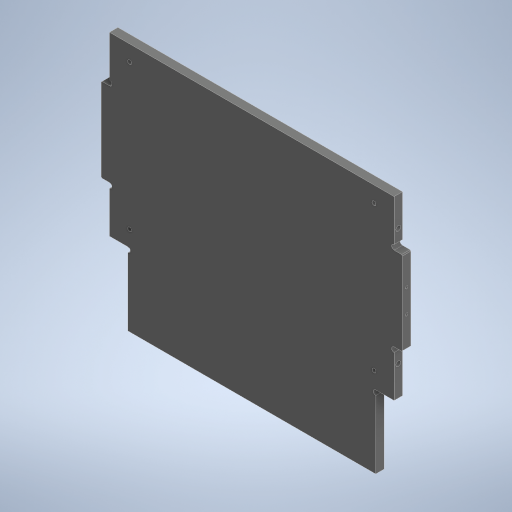
# Autodesk Inventor part: TorsoCoverFrameBasis
Saved by Autodesk Inventor 2024.2 (Build 282272000, 272)
## iProperties
Created: 2024-01-05
Part Number: TorsoCoverFrameBasis
Material: Acetal Resin, Black
Document SubType Name: Modeling
Designer: Masato Kubotera
Density: 1.425 g/cm^3
Appearance: Gray
Vendor: meviy
Mass: 132.259 g
Surface Area: 403.156 cm^2
Volume: 92.813 cm^3
Author: Masato Kubotera
Autodesk Inventor part; units mm, degrees
ref_plane "YZ Plane" through (0, 0, 0) normal (1, 0, 0) x (0, 1, 0)
ref_plane "XZ Plane" through (0, 0, 0) normal (0, 1, 0) x (-1, 0, 0)
ref_plane "XY Plane" through (0, 0, 0) normal (0, 0, 1) x (1, 0, 0)
sketch "Sketch1" plane through (0, 0, 0) normal (1, 0, 0) x (0, 1, 0)
  line L0 (-90, 74.5) -> (90, 74.5)
  line L1 (90, 74.5) -> (90, -74.5)
  line L2 (90, -74.5) -> (-90, -74.5)
  line L3 (-90, -74.5) -> (-90, 74.5) construction
  line L4 (-90, 74.5) -> (90, -74.5) construction
  line L5 (90, 74.5) -> (-90, -74.5) construction
  line L6 (85, 74.5) -> (85, 46.75)
  line L7 (85, 46.75) -> (90, 46.75)
  line L8 (0, 74.5) -> (0, -74.5)
  line L9 (90, 0) -> (-90, 0) construction
  arc A0 (85, 49.75) -> (85, 46.75) centre (85, 48.25) ccw
  line L10 (-90, 74.5) -> (-90, -74.5)
  circle A1 centre (73, 65) radius 3 construction
  arc A2 (73, 67.1) -> (73, 62.9) centre (73, 65) ccw construction
  line L11 (73, 67.1) -> (76.5201, 67.1) construction
  arc A3 (76.5201, 62.9) -> (76.5201, 67.1) centre (80.5, 65) ccw construction
  line L12 (73, 65) -> (80.5, 65) construction
  line L13 (73, 62.9) -> (76.5201, 62.9) construction
  line L14 (90, 28.75) -> (85, 28.75) construction
  line L15 (90, 14.75) -> (85, 14.75) construction
  line L16 (90, 21.75) -> (85, 21.75) construction
  line L17 (85, -3.25) -> (90, -3.25)
  arc A4 (85, -3.25) -> (85, -6.25) centre (85, -4.75) ccw
  line L18 (85, -6.25) -> (85, -74.5)
  line L19 (90, -31) -> (-90, -31)
  line L20 (74, -31) -> (74, -74.5)
  line L21 (-90, 21.75) -> (90, 21.75) construction
  circle A5 centre (73, -21.5) radius 3 construction
  arc A6 (73, -19.4) -> (73, -23.6) centre (73, -21.5) ccw construction
  line L22 (73, -23.6) -> (76.5201, -23.6) construction
  arc A7 (76.5201, -23.6) -> (76.5201, -19.4) centre (80.5, -21.5) ccw construction
  line L23 (73, -21.5) -> (80.5, -21.5) construction
  line L24 (73, -19.4) -> (76.5201, -19.4) construction
  arc A8 (74, -31) -> (74, -34) centre (74, -32.5) ccw
  point P0 (0, 0)
  point P1 (90, -3.25)
  point P2 (85, -31)
  point P3 (85, 65)
  point P4 (85, -21.5)
  point P5 (0, -31)
  dimension "d0" = 180
  dimension "d1" = 149
  dimension "d2" = 1.5
  dimension "d3" = 5
  dimension "d15" = 6
  dimension "d16" = 4.2
  dimension "d17" = 9
  dimension "d18" = 5
  dimension "d27" = 5
  dimension "d28" = 14
  dimension "d38" = 50
  dimension "d40" = 52.75
  dimension "d44" = 11
  dimension "d45" = 43.5
  dimension "d46" = 5
  dimension "d47" = 105.5
  constraints: 48 end point, 15 point on circle, 14 symmetric about line, 10 horizontal, 10 point on line, 9 centre point, 5 midpoint, 4 coincident, 4 tangent, 2 vertical, 1 collinear, 1 equal radius, 1 parallel, 1 perpendicular, 17 other
  measures "d0" distance of L2.start L2.end
  measures "d1" distance of L0.end L2.start
  measures "d2" radius of A0
  measures "d15" diameter of A1
  measures "d16" diameter of A2
  measures "d17" diameter of A3
  measures "d18" distance edge to line of A3 L0
  measures "d27" distance of L14.start L14.end
  measures "d28" distance of L15.start L14.start
  measures "d38" distance of L17.end L7.end
  measures "d40" distance between parallel lines of L0 L16
  measures "d44" distance between parallel lines of L20 L18
  measures "d45" distance of L20.start L20.end
  measures "d47" distance of L19.start L0.end
extrude "Extrusion1" add sketch "Sketch1" along normal blind 5 contours L0 L6 A0 L7 L1 L17 A4 L18 L19 L8 | L19 A8 L20 L2 L8
sketch "Sketch2" plane through (0, 90, 46.75) normal (0, 1, 0) x (1, 0, 0)
  line L0 (5, 32) -> (0, 32) construction
  line L1 (5, 18) -> (0, 18) construction
  line L2 (5, 50) -> (5, 0) projected
  line L3 (0, 50) -> (0, 0) projected
  point P0 (0, 46.75)
  point P1 (2.5, 32)
  point P2 (2.5, 18)
  point P3 (0, 18)
  point P4 (0, 32)
  point P5 (5, 121.25)
  point P6 (5, -27.75)
  point P7 (0, 121.25)
  point P8 (0, -27.75)
  point P9 (5, 77.75)
  point P10 (0, 77.75)
  constraints: 4 end point, 2 horizontal, 2 midpoint, 2 point on line, 1 other
hole "Side-M2" at (2.5, 90, 14.75) at (2.5, 90, 28.75) direction (0, -1, 0) diameter 1.567 depth 5 thread size "M2x0.4" class "6H" standard "ANSI Metric M Profile"
hole "M3" at (0, 73, 65) at (0, 73, -21.5) direction (1, 0, 0) diameter 2.459 end through all thread size "M3x0.5" class "6H" standard "ANSI Metric M Profile"
sketch "Sketch3" plane through (0, 85, 74.5) normal (0, 1, 0) x (1, 0, 0)
  line L0 (5, 24.75) -> (5, 0) projected
  line L1 (5, 17.75) -> (0, 17.75)
  line L2 (5, 105.5) -> (5, 80.75) projected
  line L3 (5, 87.75) -> (0, 87.75)
  line L4 (0, 24.75) -> (0, 0) projected
  line L5 (0, 105.5) -> (0, 80.75) projected
  line L6 (0, 52.75) -> (5, 52.75) construction
  point P0 (0, 74.5)
  point P1 (2.5, 17.75)
  point P2 (2.5, 87.75)
  point P3 (0, 52.75)
  dimension "d48" = 70
  constraints: 6 end point, 5 point on line, 3 horizontal, 2 midpoint, 1 symmetric about line
  measures "d48" distance of point (2.5, 87.75) point (2.5, 17.75)
hole "Phi3.0" at (2.5, 85, 56.75) at (2.5, 85, -13.25) direction (0, -1, 0) diameter 3 depth 6
chamfer "C0.5" distance 0.5 angle 45 2 edges at (2.5, 90, 46.75) (2.5, 90, -3.25)
mirror "Mirror1" about plane through (0, 0, 0) normal (0, 1, 0)
equation "\"d40\" = 0.5 * d47"
equation "\"d13\" = d27"
body "Solid1"
